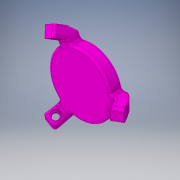
# Autodesk Inventor part: BottomPlatform
Saved by Autodesk Inventor 2019 (Build 230136000, 136)
## iProperties
Created: 2022-07-06
Part Number: BottomPlatform
Material: Generic
Document SubType Name: Modeling
Designer: zreik
Density: 1 g/cm^3
Appearance: Magenta
Author: zreik
Autodesk Inventor part; units mm, degrees
ref_plane "YZ Plane" through (0, 0, 0) normal (1, 0, 0) x (0, 1, 0)
ref_plane "XZ Plane" through (0, 0, 0) normal (0, 1, 0) x (-1, 0, 0)
ref_plane "XY Plane" through (0, 0, 0) normal (0, 0, 1) x (1, 0, 0)
sketch "Sketch1" plane through (0, 0, 0) normal (0, 0, 1) x (1, 0, 0)
  circle A0 centre (0, 0) radius 25
  line L0 (15, -5) -> (35, -5)
  line L1 (35, -5) -> (35, 5)
  line L2 (35, 5) -> (15, 5)
  line L3 (15, 5) -> (15, -5)
  line L4 (15, -5) -> (35, 5) construction
  line L5 (35, -5) -> (15, 5) construction
  point P0 (25, 0)
  dimension "d0" = 50
  dimension "d3" = 10
  dimension "d4" = 20
  dimension "d5" = 0
  constraints: 12 end point, 2 midpoint, 2 parallel, 1 coincident, 1 horizontal, 1 horizontal alignment, 1 perpendicular, 2 other
  measures "d3" distance of L0.end L1.end
  measures "d4" distance of L0.start L0.end
  measures "d5" vertical distance of point (0, 0) point (25, 0)
extrude "Extrusion1" add sketch "Sketch1" along normal mid plane 10 contours A0 L0 L3 L2 | L2 L3 L0 A0
extrude "Extrusion2" add sketch "Sketch1" along normal mid plane 10 contours A0 L0 L3 L2 | A0 L2 L1 L0 picked at (18.3333, 0)
chamfer "Chamfer1" distance 7 angle 30 1 edges at (35, 0, 5) measured on face at (34.5, 0, 5)
sketch "Sketch2" plane through (28, -5, 5) normal (0.5, 0, 0.8660254) x (0.8660254, 0, -0.5)
  line L0 (8.0829, 0) -> (0, 0)
  line L1 (0, 0) -> (0, 10)
  line L2 (0, 10) -> (8.0829, 10)
  line L3 (8.0829, 10) -> (8.0829, 0)
  line L4 (8.0829, 0) -> (0, 10) construction
  line L5 (0, 0) -> (8.0829, 10) construction
  line L6 (0, 10) -> (0, 0) projected
  line L7 (8.0829, 0) -> (8.0829, 10) projected
  line L8 (8.0829, 10) -> (0, 10) projected
  line L9 (0, 0) -> (8.0829, 0) projected
  point P0 (-21.7487, 5)
  point P1 (4.0415, 5)
  dimension "d11" = 0
  dimension "d12" = 0
  dimension "d13" = 0
  dimension "d14" = 0
  constraints: 12 end point, 2 midpoint, 2 parallel, 1 horizontal, 1 perpendicular
  measures "d11" distance between parallel lines of L1 L6
  measures "d12" distance between parallel lines of L7 L3
  measures "d13" distance between parallel lines of L8 L2
  measures "d14" distance between parallel lines of L9 L0
extrude "Extrusion3" add sketch "Sketch2" along normal blind 10
sketch "Sketch3" plane through (28, -5, 5) normal (-0.8660254, 0, 0.5) x (0.5, 0, 0.8660254)
  circle A0 centre (5, 5) radius 3.5
  line L0 (10, 10) -> (10, 0) projected
  line L1 (0, 10) -> (0, 0) projected
  line L2 (0, 0) -> (10, 0) projected
  line L3 (0, 10) -> (10, 10) projected
  point P0 (-18.3301, 5)
  dimension "d17" = 7
  dimension "d18" = 5
  dimension "d19" = 5
  dimension "d20" = 5
  dimension "d21" = 5
  constraints: 1 centre point
  measures "d17" diameter of A0
  measures "d18" distance from line of L0 A0.centre
  measures "d19" distance from line of L1 A0.centre
  measures "d20" distance from line of L2 A0.centre
  measures "d21" distance from line of L3 A0.centre
extrude "Extrusion5" cut sketch "Sketch3" against normal blind 3 contours A0
sketch "Sketch4" plane through (33.0981, 0, 7.8301) normal (-0.8660254, 0, 0.5) x (0.5, 0, 0.8660254)
  circle A0 centre (0, 0) radius 2.5
  circle A1 centre (0, 0) radius 3.5 projected
  point P0 (-23.3301, 0)
  dimension "d32" = 5
  constraints: 1 centre point, 1 concentric
  measures "d32" diameter of A0
extrude "Extrusion6" cut sketch "Sketch4" against normal through all contours A0
chamfer "Chamfer3" distance 5.5 angle 45 1 edges at (35, 0, -5)
sketch "Sketch5" plane through (35, -5, 0.9585) normal (0.8660254, 0, -0.5) x (-0.5, 0, -0.8660254)
  circle A0 centre (-5, 5) radius 3.5
  circle A1 centre (-5, 5) radius 2.5 projected
  point P0 (18.3301, 5)
  dimension "d35" = 7
  constraints: 1 centre point, 1 concentric
  measures "d35" diameter of A0
extrude "Extrusion7" cut sketch "Sketch5" against normal blind 3
pattern_circular "Circular Pattern1" count 3 over 360 about axis through (0, 0, 0) along (0, 0, 1) of "Extrusion3", "Extrusion2", "Chamfer1", "Extrusion5", "Extrusion6", "Extrusion7", "Chamfer3"
fillet "Fillet1" radius 2 12 edges at (-14, -24.2487, 5) (-14, 24.2487, 5) (28, 0, 5) (24.4949, -5, 0) (-7.9173, -23.7132, 0) (-16.5776, -18.7132, 0) (-16.5776, 18.7132, 0) (24.4949, 5, 0) (-7.9173, 23.7132, 0) (29.5, 0, -5) (-14.75, 25.5477, -5) (-14.75, -25.5477, -5)
fillet "Fillet2" radius 2 60 edges at (-22.5801, 29.1099, 11.6395) (-13.9199, 34.1099, 11.6395) (36.5, -5, 11.6395) (36.5, 5, 11.6395) (27.8453, -5, 5.2679) (26.4611, -5, 5) (24.8596, -5.413, 5) (12.5, -21.6506, 5) (-7.742, -24.2356, 5) (-8.9004, -25.4159, 5) (-9.5925, -26.6147, 5.2679) (-11.0642, -29.1638, 9.8301) (30.7887, -5, 9.8301) (-7.742, 24.2356, 5) (-8.9004, 25.4159, 5) (-9.5925, 26.6147, 5.2679) (-11.0642, 29.1638, 9.8301) (24.8596, 5.413, 5) (26.4611, 5, 5) (27.8453, 5, 5.2679) (30.7887, 5, 9.8301) (12.5, 21.6506, 5) (-17.1176, -18.8226, 5) (-17.5607, -20.4159, 5) (-18.2528, -21.6147, 5.2679) (-19.7245, -24.1638, 9.8301) (-17.1176, 18.8226, 5) (-17.5607, 20.4159, 5) (-18.2528, 21.6147, 5.2679) (-19.7245, 24.1638, 9.8301) (-25, 0, 5) (-7.742, -24.2356, -5) (-9.357, -26.2067, -5) (-10.3883, -27.9931, -4.8478) (-11.9413, -30.683, -1.9571) (24.8596, -5.413, -5) (27.3742, -5, -5) (29.4369, -5, -4.8478) (32.5429, -5, -1.9571) (12.5, -21.6506, -5) (-13.9199, -34.1099, 11.6395) (-22.5801, -29.1099, 11.6395) (-17.1176, 18.8226, -5) (-18.0172, 21.2067, -5) (-19.0486, 22.9931, -4.8478) (-20.6016, 25.683, -1.9571) (-17.1176, -18.8226, -5) (-18.0172, -21.2067, -5) (-19.0486, -22.9931, -4.8478) (-20.6016, -25.683, -1.9571) (-25, 0, -5) (24.8596, 5.413, -5) (27.3742, 5, -5) (29.4369, 5, -4.8478) (32.5429, 5, -1.9571) (-7.742, 24.2356, -5) (-9.357, 26.2067, -5) (-10.3883, 27.9931, -4.8478) (-11.9413, 30.683, -1.9571) (12.5, 21.6506, -5)
equation "\"d18\" = d19"
equation "\"d20\" = d21"
body "Solid1"
